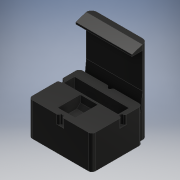
# Autodesk Inventor part: SMF3300_CONECTOR
Saved by Autodesk Inventor 2018 (Build 220112000, 112)
## iProperties
Created: 2020-08-07
Part Number: SMF3300_CONECTOR
Material: Generic
Document SubType Name: Modeling
Designer: sawer
Density: 1 g/cm^3
Appearance: Glossy - Black
Author: sawer
Autodesk Inventor part; units mm, degrees
note: some values were not read from the file. Chosen so that the rebuilt part matches the saved one: second side of "Extrusion1".
ref_plane "YZ Plane" through (0, 0, 0) normal (1, 0, 0) x (0, 1, 0)
ref_plane "XZ Plane" through (0, 0, 0) normal (0, 1, 0) x (-1, 0, 0)
ref_plane "XY Plane" through (0, 0, 0) normal (0, 0, 1) x (1, 0, 0)
sketch "Sketch1" plane through (0, 0, 0) normal (0, 0, 1) x (1, 0, 0)
  line L0 (0, 0) -> (9, 0) construction
  line L1 (9, 0) -> (9, 7.2)
  line L2 (9, 7.2) -> (-9, 7.2)
  line L3 (-9, 7.2) -> (-9, -7.2)
  line L4 (-9, -7.2) -> (9, -7.2)
  line L5 (9, -7.2) -> (9, 0)
  line L6 (9, -7.2) -> (9, 3.05) construction
  dimension "d0" = 9
  dimension "d1" = 7.2
  dimension "d2" = 18
  dimension "d3" = 14.4
  dimension "d4" = 18
  constraints: 14 end point, 3 perpendicular, 1 horizontal, 1 point on line, 1 vertical
  measures "d0" distance of L0.start L0.end
  measures "d1" distance of L0.end L1.end
  measures "d2" distance of L1.end L2.end
  measures "d3" distance of L2.end L3.end
  measures "d4" distance of L3.end L4.end
extrude "Extrusion1" add sketch "Sketch1" along normal blind 9.5
fillet "Fillet1" radius 1 4 edges at (9, 7.2, 4.75) (9, -7.2, 4.75) (-9, -7.2, 4.75) (-9, 7.2, 4.75)
sketch "Sketch3" plane through (0, 0, 9.5) normal (0, 0, 1) x (1, 0, 0)
  line L0 (-9, 6.2) -> (-9, -6.2) projected
  line L1 (9, -6.2) -> (9, 6.2) projected
  line L2 (8, 7.2) -> (-8, 7.2) projected
  line L3 (0, 7.2) -> (0.5, 7.2)
  line L4 (0.5, 7.2) -> (0.5, 6.825)
  line L5 (0.125, 6.45) -> (-0.125, 6.45)
  line L6 (-0.5, 6.825) -> (-0.5, 7.2)
  line L7 (8, -7.2) -> (-8, -7.2) projected
  line L8 (0, -7.2) -> (-0.5, -7.2)
  line L9 (-0.5, -7.2) -> (-0.5, -6.825)
  line L10 (-0.125, -6.45) -> (0.125, -6.45)
  line L11 (0.5, -6.825) -> (0.5, -7.2)
  line L12 (0.5, -7.2) -> (0, -7.2)
  line L13 (-0.125, 7.2) -> (0, 7.2)
  arc A0 (0.125, 6.45) -> (0.5, 6.825) centre (0.125, 6.825) ccw
  arc A1 (-0.5, 6.825) -> (-0.125, 6.45) centre (-0.125, 6.825) ccw
  arc A2 (0.5, -6.825) -> (0.125, -6.45) centre (0.125, -6.825) ccw
  arc A3 (-0.125, -6.45) -> (-0.5, -6.825) centre (-0.125, -6.825) ccw
  line L14 (0, -6.45) -> (0, -6.132) construction
  line L15 (8, 7.2) -> (9, 7.2) construction
  line L16 (9, 7.2) -> (9, 6.2) construction
  line L17 (9, 7.2) -> (9, 2.2) construction
  line L18 (9, 2.2) -> (8.5, 2.2)
  line L19 (8, 1.7) -> (8, 1.7)
  line L20 (8.5, 1.2) -> (9, 1.2)
  arc A4 (8.5, 2.2) -> (8, 1.7) centre (8.5, 1.7) ccw
  arc A5 (8, 1.7) -> (8.5, 1.2) centre (8.5, 1.7) ccw
  line L21 (-8, 7.2) -> (-9, 7.2) construction
  line L22 (-9, 7.2) -> (-9, 6.2) construction
  line L23 (-9, 7.2) -> (-9, 2.2) construction
  line L24 (-9, 2.2) -> (-8.5, 2.2)
  line L25 (-8, 1.7) -> (-8, 1.7)
  line L26 (-8.5, 1.2) -> (-9, 1.2)
  arc A6 (-8, 1.7) -> (-8.5, 2.2) centre (-8.5, 1.7) ccw
  arc A7 (-8.5, 1.2) -> (-8, 1.7) centre (-8.5, 1.7) ccw
  line L27 (-9, 1.2) -> (-9, 2.2)
  line L28 (9, 1.2) -> (9, 2.2)
  line L29 (-0.125, 7.2) -> (-0.5, 7.2)
  point P0 (0, 0)
  point P1 (0.5, 6.45)
  point P2 (-0.5, 6.45)
  point P3 (-8, -7.2)
  point P4 (8, -7.2)
  point P5 (-0.5, -6.45)
  point P6 (0.5, -6.45)
  point P7 (8, 2.2)
  point P8 (8, 1.2)
  point P9 (-8, 2.2)
  point P10 (-8, 1.2)
  dimension "d70" = 0.5
  dimension "d71" = 0.75
  dimension "d72" = 1
  dimension "d73" = 0.5
  dimension "d74" = 0.75
  dimension "d75" = 1
  dimension "d76" = 0.75
  dimension "d92" = 5
  dimension "d93" = 1
  dimension "d94" = 1
  dimension "d96" = 5
  dimension "d97" = 1
  dimension "d98" = 1
  constraints: 52 end point, 20 point on line, 17 point on circle, 16 tangent, 11 perpendicular, 8 centre point, 6 horizontal, 5 equal radius, 2 vertical, 1 midpoint, 1 parallel, 8 other
  measures "d70" distance of L3.start L3.end
  measures "d71" distance of L3.end point (0.5, 6.45)
  measures "d72" distance of point (0.5, 6.45) point (-0.5, 6.45)
  measures "d73" distance of L8.start L8.end
  measures "d74" distance of L8.end point (-0.5, -6.45)
  measures "d75" distance of point (-0.5, -6.45) point (0.5, -6.45)
  measures "d76" distance of point (0.5, -6.45) L11.end
  measures "d92" distance of L15.end L17.end
  measures "d93" distance of L17.end point (8, 2.2)
  measures "d94" distance of point (8, 2.2) point (8, 1.2)
  measures "d96" distance of L21.end L23.end
  measures "d97" distance of L23.end point (-8, 2.2)
  measures "d98" distance of point (-8, 2.2) point (-8, 1.2)
extrude "Extrusion3" cut sketch "Sketch3" against normal blind 2.5
fillet "Fillet5" radius 0.5 8 edges at (9, 2.2, 8.25) (0.5, -7.2, 8.25) (-0.5, -7.2, 8.25) (9, 1.2, 8.25) (-9, 2.2, 8.25) (-9, 1.2, 8.25) (0.5, 7.2, 8.25) (-0.5, 7.2, 8.25)
sketch "Sketch6" plane through (0, 0, 9.5) normal (0, 0, 1) x (1, 0, 0)
  line L0 (0, 0) -> (0, 1) construction
  line L1 (1.75, -4.45) -> (-1.75, -4.45) construction
  line L2 (0, -4.45) -> (0, -5.45) construction
  line L3 (0, -5.45) -> (2.5, -5.45)
  line L4 (2.5, -5.45) -> (2.5, 1)
  line L5 (2.5, 1) -> (0, 1)
  line L6 (0, 1) -> (-2.5, 1)
  line L7 (-2.5, 1) -> (-2.5, -5.45)
  line L8 (-2.5, -5.45) -> (0, -5.45)
  dimension "d103" = 1
  dimension "d104" = 1
  dimension "d105" = 2.5
  dimension "d106" = 2.5
  constraints: 16 end point, 4 perpendicular, 2 horizontal, 2 vertical, 1 midpoint
  measures "d103" distance of L0.start L0.end
  measures "d104" distance of L2.start L2.end
  measures "d105" distance of L2.end L3.end
  measures "d106" distance of L0.end L6.end
extrude "Extrusion5" cut sketch "Sketch6" against normal blind 3
chamfer "Chamfer2" distance 1 angle 45 1 edges at (0, 1, 6.5)
chamfer "Chamfer3" distance 1 angle 45 1 edges at (0, -5.45, 6.5)
sketch "Sketch7" plane through (0, 0, 9.5) normal (0, 0, 1) x (1, 0, 0)
  line L0 (0, 0) -> (0, 1.5) construction
  line L1 (0, 1.5) -> (7.75, 1.5)
  line L2 (7.75, 1.5) -> (7.75, 4.6)
  line L3 (7.75, 4.6) -> (-7.75, 4.6)
  line L4 (-7.75, 4.6) -> (-7.75, 1.5)
  line L5 (-7.75, 1.5) -> (0, 1.5)
  dimension "d118" = 1.5
  dimension "d119" = 7.75
  dimension "d120" = 3.1
  dimension "d121" = 15.5
  constraints: 12 end point, 5 perpendicular, 1 point on line, 1 vertical
  measures "d118" distance of L0.start L0.end
  measures "d119" distance of L0.end L1.end
  measures "d120" distance of L1.end L2.end
  measures "d121" distance of L2.end L3.end
extrude "Extrusion6" cut sketch "Sketch7" against normal up to surface (9.5 mm away)
chamfer "Chamfer4" distance 1.5 angle 45 2 edges at (0, 1.5, 0) (0, 4.6, 0)
sketch "Sketch9" plane through (-8, 7.2, 0) normal (0, 1, 0) x (1, 0, 0)
  line L0 (7.875, -7) -> (8.125, -7) construction
  line L1 (8, -7) -> (8, 0) construction
  line L2 (0, 0) -> (16, 0) projected
  line L3 (8, 0) -> (16, 0)
  line L4 (16, 0) -> (16, -7)
  line L5 (16, -9.5) -> (16, 0) projected
  line L6 (16, -7) -> (0, -7)
  line L7 (0, 0) -> (0, -9.5) projected
  line L8 (0, -7) -> (0, 0)
  line L9 (0, 0) -> (8, 0)
  dimension "d128" = 7
  dimension "d129" = 16
  constraints: 12 end point, 2 point on line, 1 horizontal, 1 midpoint, 1 perpendicular, 1 vertical
  measures "d128" distance of L2.end L4.end
  measures "d129" distance of L4.end L6.end
extrude "Extrusion7" add sketch "Sketch9" along normal blind 2.5
fillet "Fillet6" radius 1.5 2 edges at (8, 9.7, 3.5) (-8, 9.7, 3.5)
sketch "Sketch10" plane through (0, 0, 7) normal (0, 0, 1) x (1, 0, 0)
  line L0 (-8, 7.2) -> (-8, 8.2) projected
  line L1 (-8, 8.2) -> (8, 8.2)
  line L2 (-6.5, 9.7) -> (6.5, 9.7) projected
  line L3 (0, 9.7) -> (-6.5, 9.7)
  line L4 (-8, 8.2) -> (-8, 8.2)
  arc A0 (-6.5, 9.7) -> (-8, 8.2) centre (-6.5, 8.2) ccw
  line L5 (0, 9.7) -> (6.5, 9.7)
  line L6 (8, 8.2) -> (8, 8.2)
  arc A1 (8, 8.2) -> (6.5, 9.7) centre (6.5, 8.2) ccw
  point P0 (0, 0)
  point P1 (-8, 9.7)
  point P2 (8, 9.7)
  dimension "d133" = 16
  dimension "d134" = 8
  dimension "d135" = 1.5
  dimension "d136" = 8
  dimension "d137" = 1.5
  constraints: 10 end point, 4 point on circle, 4 point on line, 4 tangent, 2 centre point, 2 horizontal, 1 collinear, 1 midpoint
  measures "d133" distance of L0.end L1.end
  measures "d134" distance of L3.start point (-8, 9.7)
  measures "d135" radius of A0
  measures "d136" distance of L3.start point (8, 9.7)
  measures "d137" radius of A1
extrude "Extrusion8" add sketch "Sketch10" along normal blind 16.5
sketch "Sketch11" plane through (-8, 8.2, 7) normal (0, -1, 0) x (1, 0, 0)
  line L0 (0, 0) -> (0, 16.5) projected
  line L1 (0, 16.5) -> (0, 15)
  line L2 (0, 15) -> (16, 15)
  line L3 (16, 0) -> (16, 16.5) projected
  line L4 (16, 15) -> (16, 16.5)
  line L5 (16, 16.5) -> (0, 16.5)
  point P0 (8, -7)
  dimension "d140" = 1.5
  dimension "d141" = 16
  constraints: 8 end point, 2 point on line, 1 perpendicular
  measures "d140" distance of L0.end L1.end
  measures "d141" distance of L1.end L2.end
extrude "Extrusion9" add sketch "Sketch11" along normal blind 3
chamfer "Chamfer5" distance 1 distance2 3 1 edges at (0, 5.2, 23.5) measured on face at (-2.6667, 5.2, 23)
chamfer "Chamfer6" distance 0.5 distance2 5 1 edges at (0, 8.2, 7) measured on face at (-0.3303, 7.8667, 7)
body "Solid1"
